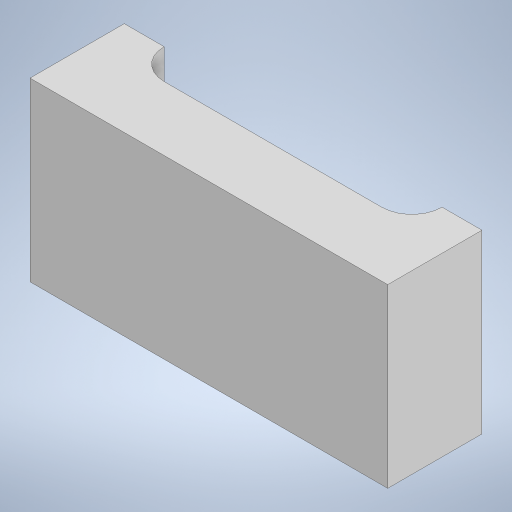
# Autodesk Inventor part: drzak_kable_guma
Saved by Autodesk Inventor 2023 (Build 270158000, 158)
## iProperties
Created: 2025-01-22
Part Number: drzak_kable_guma
Material: Všeobecné
Document SubType Name: Modeling
Designer: lisnik
Density: 1 g/cm^3
Appearance: Výchozí
Author: lisnik
Autodesk Inventor part; units mm, degrees
ref_plane "YZ Plane" through (0, 0, 0) normal (1, 0, 0) x (0, 1, 0)
ref_plane "XZ Plane" through (0, 0, 0) normal (0, 1, 0) x (-1, 0, 0)
ref_plane "XY Plane" through (0, 0, 0) normal (0, 0, 1) x (1, 0, 0)
sketch "Náčrt1" plane through (0, 0, 0) normal (0, 0, 1) x (1, 0, 0)
  line L0 (-20.72, 0) -> (20.72, 0) projected
  line L1 (0, -10.22) -> (0, 10.22) projected
  line L2 (-14.8, 7.3) -> (14.8, 7.3)
  line L3 (14.8, 7.3) -> (14.8, -7.3)
  line L4 (14.8, -7.3) -> (-14.8, -7.3)
  line L5 (-14.8, -7.3) -> (-14.8, 7.3)
  point P0 (0, 0)
  point P1 (0, 7.3)
  point P2 (14.8, 0)
  dimension "d0" = 29.6
  dimension "d1" = 14.6
  constraints: 8 end point, 2 midpoint, 2 parallel, 2 point on line, 1 horizontal, 1 perpendicular
  measures "d0" distance of L3.end L4.end
  measures "d1" distance of L2.end L3.end
extrude "Vysunutí1" add sketch "Náčrt1" along normal blind 7.8
sketch "Náčrt2" plane through (-14.8, -7.3, 0) normal (0, -1, 0) x (1, 0, 0)
  line L0 (0, 0) -> (29.6, 0) projected
  line L1 (29.6, 0) -> (29.6, 7.8) projected
  line L2 (0, 7.8) -> (29.6, 7.8) projected
  line L3 (0, 0) -> (0, 7.8) projected
  point P0 (14.8, 0)
  point P1 (14.8, 0)
  constraints: 1 midpoint
hole "Díra1" at (0, -7.3, 0) direction (0, 1, 0) diameter 5 end through all
sketch "Náčrt3" plane through (-14.8, -7.3, 7.8) normal (0, -1, 0) x (1, 0, 0)
  line L0 (5.8, -7.8) -> (23.8, -7.8) construction
  line L1 (17.3, -7.8) -> (29.6, -7.8) projected
  line L2 (5.8, -10.3) -> (23.8, -10.3)
  line L3 (23.8, -5.3) -> (5.8, -5.3)
  arc A0 (5.8, -5.3) -> (5.8, -10.3) centre (5.8, -7.8) ccw
  arc A1 (23.8, -10.3) -> (23.8, -5.3) centre (23.8, -7.8) ccw
  point P0 (14.8, -7.8)
  dimension "d14" = 9
  dimension "d15" = 2.5
  constraints: 8 end point, 4 point on circle, 4 tangent, 2 centre point, 1 midpoint, 1 parallel, 1 point on line
  measures "d14" distance of point (14.8, -7.8) L0.end
  measures "d15" distance between parallel lines of L0 L3
extrude "Vysunutí2" cut sketch "Náčrt3" against normal through all
